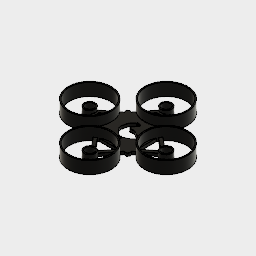
tiny-whoop-redesign (Autodesk Fusion 360 design; units mm, degrees)
Autodesk Fusion 360 part; units mm, degrees
note: some values were not read from the file. Chosen so that the rebuilt part matches the saved one: which bodies a step acts on; which face or edge a step refers to; a direction. Set by a fixed rule: which sketch regions a step uses.
sketch "Sketch1" plane through (0, 0, 0) normal (0, 1, 0) x (1, 0, 0)
  line L0 (-13.5, -13.5) -> (13.5, -13.5)
  line L1 (13.5, -13.5) -> (13.5, 13.5)
  line L2 (13.5, 13.5) -> (-13.5, 13.5)
  line L3 (-13.5, 13.5) -> (-13.5, -13.5)
  line L4 (-13.5, -13.5) -> (13.5, 13.5) construction
  line L5 (13.5, -13.5) -> (-13.5, 13.5) construction
  circle A0 centre (0, 30.8) radius 16.3
  circle A1 centre (0, 30.8) radius 3.5
  circle A2 centre (-13.5, 13.5) radius 2
  line L6 (0, 30.8) -> (13.5, 13.5)
  line L7 (0, 30.8) -> (-13.5, 13.5)
  dimension "d1" = 27
  dimension "d4" = 7
  dimension "d5" = 4
  dimension "d21" = 17.3
  dimension "d22" = 32.6
  dimension "d23" = 27
  measures "d1" distance of L0.end L1.end
  measures "d4" diameter of A1
  measures "d5" diameter of A2
  measures "d21" distance of L2 A0.centre
  measures "d22" diameter of A0
  measures "d23" distance of L1 L3
surface "Extrude1" add extruded along (0, 1, 0) between 0 and 10 path "Sketch1" along A0 makes body 1
surface "Extrude2" add extruded along (0, 1, 0) between 0 and 5 path "Sketch1" along A1 separate body makes body 2
extrude "Extrude3" add sketch "Sketch1" along normal blind 2.5 separate body contours L2 A0 A2 L6 L7 | L2 A2 L7 | A0 A1 L6 L7 picked at (6.7383, 20.8692) makes body 3
shell "Shell1" thickness 2.5 removed faces 2 at (-0.0858, 2.5, -21.0695) at (-0.0858, 0, -21.0695) on bodies 3
thicken "Thicken1" add thickness -1 1 faces at (16.2797, 6.6667, -29.9875) separate body on bodies 1 makes body 4
thicken "Thicken2" add thickness -1 1 faces at (3.4956, 3.3333, -30.6255) separate body on bodies 2 makes body 5
delete_body "RemoveBody1" bodies 2
delete_body "RemoveBody2" bodies 1
extrude "Extrude4" add sketch "Sketch1" along normal blind 2.5 contours L3 A2 L7 | L2 L3 A2 bodies 3
pattern_circular "C-Pattern1" count 4 over 360 about axis through (0, 1.75, 0) along (0, 1, 0) of bodies 4 5 3 makes body 6 at (-14.3333, 2.5, 2.126) makes body 7 at (2.126, 2.5, 14.3333) makes body 8 at (14.3333, 2.5, -2.126) makes body 9 at (-30.5757, 3.3333, -4.4944) makes body 10 at (-4.4944, 3.3333, 30.5757) makes body 11 at (30.5757, 3.3333, 4.4944) makes body 12 at (-29.9377, 6.6667, -17.2785) makes body 13 at (-17.2785, 6.6667, 29.9377) makes body 14 at (29.9377, 6.6667, 17.2785)
extrude "Extrude5" add sketch "Sketch1" along normal blind 2.5 contours L0 L1 L2 L3 A2 bodies 4 5 9 10 11 3 6 7 8 12 13 14
sketch "Sketch2" plane through (0, 0, 0) normal (0, -1, 0) x (1, 0, 0)
  line L0 (17.1612, 10.643) -> (15.0767, 12.2696)
  arc A0 (15.0767, 12.2696) -> (12.2696, 15.0767) centre (13.5, 13.5) ccw
  line L1 (12.2696, 15.0767) -> (10.643, 17.1612)
  arc A1 (10.643, 17.1612) -> (-10.643, 17.1612) centre (0, 30.8) ccw
  line L2 (-10.643, 17.1612) -> (-12.2696, 15.0767)
  arc A2 (-12.2696, 15.0767) -> (-15.0767, 12.2696) centre (-13.5, 13.5) ccw
  line L3 (-15.0767, 12.2696) -> (-17.1612, 10.643)
  arc A3 (-17.1612, 10.643) -> (-17.1612, -10.643) centre (-30.8, 0) ccw
  line L4 (-17.1612, -10.643) -> (-15.0767, -12.2696)
  arc A4 (-15.0767, -12.2696) -> (-12.2696, -15.0767) centre (-13.5, -13.5) ccw
  line L5 (-12.2696, -15.0767) -> (-10.643, -17.1612)
  arc A5 (-10.643, -17.1612) -> (10.643, -17.1612) centre (0, -30.8) ccw
  line L6 (10.643, -17.1612) -> (12.2696, -15.0767)
  arc A6 (12.2696, -15.0767) -> (15.0767, -12.2696) centre (13.5, -13.5) ccw
  line L7 (15.0767, -12.2696) -> (17.1612, -10.643)
  arc A7 (17.1612, -10.643) -> (17.1612, 10.643) centre (30.8, 0) ccw
  line L8 (16.5636, 7.9382) -> (24.9619, 1.3846)
  arc A8 (24.9619, 1.3846) -> (24.9619, -1.3846) centre (30.8, 0) ccw
  line L9 (24.9619, -1.3846) -> (16.5636, -7.9382)
  arc A9 (16, -6.8301) -> (16.5636, -7.9382) centre (30.8, 0) ccw
  line L10 (16, -6.8301) -> (16, 6.8301)
  arc A10 (16.5636, 7.9382) -> (16, 6.8301) centre (30.8, 0) ccw
  arc A11 (10.0278, 17.9496) -> (-10.0278, 17.9496) centre (0, 30.8) ccw
  line L11 (10.0278, 17.9496) -> (2.1532, 28.0407)
  arc A12 (-2.1532, 28.0407) -> (2.1532, 28.0407) centre (0, 30.8) ccw
  line L12 (-2.1532, 28.0407) -> (-10.0278, 17.9496)
  line L13 (-16.5636, -7.9382) -> (-24.9619, -1.3846)
  arc A13 (-24.9619, -1.3846) -> (-24.9619, 1.3846) centre (-30.8, 0) ccw
  line L14 (-24.9619, 1.3846) -> (-16.5636, 7.9382)
  arc A14 (-16, 6.8301) -> (-16.5636, 7.9382) centre (-30.8, 0) ccw
  line L15 (-16, 6.8301) -> (-16, -6.8301)
  arc A15 (-16.5636, -7.9382) -> (-16, -6.8301) centre (-30.8, 0) ccw
  arc A16 (-6.8301, -16) -> (-7.9382, -16.5636) centre (0, -30.8) ccw
  line L16 (-6.8301, -16) -> (6.8301, -16)
  arc A17 (7.9382, -16.5636) -> (6.8301, -16) centre (0, -30.8) ccw
  line L17 (7.9382, -16.5636) -> (1.3846, -24.9619)
  arc A18 (1.3846, -24.9619) -> (-1.3846, -24.9619) centre (0, -30.8) ccw
  line L18 (-1.3846, -24.9619) -> (-7.9382, -16.5636)
  line L19 (-10.0278, -17.9496) -> (-2.1532, -28.0407)
  arc A19 (2.1532, -28.0407) -> (-2.1532, -28.0407) centre (0, -30.8) ccw
  line L20 (2.1532, -28.0407) -> (10.0278, -17.9496)
  arc A20 (-10.0278, -17.9496) -> (10.0278, -17.9496) centre (0, -30.8) ccw
  arc A21 (-17.9496, 10.0278) -> (-17.9496, -10.0278) centre (-30.8, 0) ccw
  line L21 (-17.9496, 10.0278) -> (-28.0407, 2.1532)
  arc A22 (-28.0407, -2.1532) -> (-28.0407, 2.1532) centre (-30.8, 0) ccw
  line L22 (-28.0407, -2.1532) -> (-17.9496, -10.0278)
  line L23 (-7.9382, 16.5636) -> (-1.3846, 24.9619)
  arc A23 (-1.3846, 24.9619) -> (1.3846, 24.9619) centre (0, 30.8) ccw
  line L24 (1.3846, 24.9619) -> (7.9382, 16.5636)
  arc A24 (6.8301, 16) -> (7.9382, 16.5636) centre (0, 30.8) ccw
  line L25 (6.8301, 16) -> (-6.8301, 16)
  arc A25 (-7.9382, 16.5636) -> (-6.8301, 16) centre (0, 30.8) ccw
  arc A26 (17.9496, -10.0278) -> (17.9496, 10.0278) centre (30.8, 0) ccw
  line L26 (17.9496, -10.0278) -> (28.0407, -2.1532)
  arc A27 (28.0407, 2.1532) -> (28.0407, -2.1532) centre (30.8, 0) ccw
  line L27 (28.0407, 2.1532) -> (17.9496, 10.0278)
  spline S0 degree 5 poles (-2.1666, -3.1902) (-2.2131, -3.2344) (-2.2807, -3.3362) (-2.3073, -3.5283) (-2.2123, -3.8513) (-1.9615, -4.3155) (-1.6699, -4.7852) (-1.3964, -5.2241) (-1.1501, -5.6233) (-0.9149, -5.9884) (-0.6643, -6.3303) (-0.3814, -6.6536) (-0.0723, -6.9502) (0.2427, -7.212) (0.5353, -7.44) (0.7768, -7.6596) (0.9424, -7.9138) (1.0132, -8.2368) (0.9784, -8.6265) (0.8354, -9.0411) (0.5869, -9.4231) (0.2388, -9.7158) (-0.2025, -9.884) (-0.7286, -9.9113) (-1.3271, -9.795) (-1.9806, -9.5432) (-2.6636, -9.1699) (-3.3446, -8.6932) (-3.9906, -8.1336) (-4.5708, -7.5131) (-5.0603, -6.8538) (-5.445, -6.1765) (-5.7243, -5.4997) (-5.9167, -4.838) (-6.0522, -4.2019) (-6.1638, -3.5974) (-6.2798, -3.0259) (-6.416, -2.4838) (-6.5658, -1.9619) (-6.6995, -1.4465) (-6.777, -0.9226) (-6.758, -0.3764) (-6.6122, 0.2015) (-6.3322, 0.8132) (-5.9305, 1.4534) (-5.4324, 2.1115) (-4.8694, 2.7725) (-4.2726, 3.4186) (-3.6662, 4.0302) (-3.0606, 4.5878) (-2.4472, 5.0728) (-1.8059, 5.4681) (-1.1109, 5.7582) (-0.337, 5.9299) (0.5338, 5.9725) (1.5068, 5.8782) (2.5667, 5.6426) (3.6785, 5.2653) (4.7946, 4.7507) (5.8602, 4.109) (6.8204, 3.3572) (7.6253, 2.5197) (8.2363, 1.6294) (8.6327, 0.7288) (8.8165, -0.1298) (8.8216, -0.8816) (8.7036, -1.4593) (8.5198, -1.8118) (8.313, -1.9188) (8.0914, -1.8089) (7.8167, -1.5707) (7.4396, -1.3139) (6.9288, -1.1376) (6.3046, -1.0941) (5.6194, -1.1979) (4.9387, -1.4336) (4.3204, -1.7654) (3.7979, -2.145) (3.3545, -2.5209) (2.9336, -2.8453) (2.4654, -3.0801) (1.8893, -3.2034) (1.1766, -3.2154) (0.358, -3.1463) (-0.488, -3.0483) (-1.2626, -2.9819) (-1.747, -2.9997) (-2.0017, -3.071) (-2.1201, -3.146) (-2.1666, -3.1902) knots 0 0 0 0 0 0 0.01176471 0.02352941 0.03529412 0.04705882 0.05882353 0.07058824 0.08235294 0.09411765 0.10588235 0.11764706 0.12941176 0.14117647 0.15294118 0.16470588 0.17647059 0.18823529 0.2 0.21176471 0.22352941 0.23529412 0.24705882 0.25882353 0.27058824 0.28235294 0.29411765 0.30588235 0.31764706 0.32941176 0.34117647 0.35294118 0.36470588 0.37647059 0.38823529 0.4 0.41176471 0.42352941 0.43529412 0.44705882 0.45882353 0.47058824 0.48235294 0.49411765 0.50588235 0.51764706 0.52941176 0.54117647 0.55294118 0.56470588 0.57647059 0.58823529 0.6 0.61176471 0.62352941 0.63529412 0.64705882 0.65882353 0.67058824 0.68235294 0.69411765 0.70588235 0.71764706 0.72941176 0.74117647 0.75294118 0.76470588 0.77647059 0.78823529 0.8 0.81176471 0.82352941 0.83529412 0.84705882 0.85882353 0.87058824 0.88235294 0.89411765 0.90588235 0.91764706 0.92941176 0.94117647 0.95294118 0.96470588 0.97647059 0.98823529 1 1 1 1 1 1
  line L28 (-2.316, -9.3468) -> (-2.5138, -10.5027)
  line L29 (-2.5138, -10.5027) -> (-1.6191, -9.6681)
  line L30 (-0.743, 10.2464) -> (-0.1832, 5.9127)
  line L31 (-0.743, 10.2464) -> (-1.6827, 10.7991)
  line L32 (-1.6827, 10.7991) -> (-1.8453, 10.5227)
  line L33 (-1.8453, 10.5227) -> (-2.0079, 10.2464)
  line L34 (-2.0079, 10.2464) -> (-1.5408, 10.3846)
  line L35 (-1.5408, 10.3846) -> (-1.0317, 10.1717)
  line L36 (-1.0317, 10.1717) -> (-0.918, 5.7789)
  line L37 (0.6389, 5.9355) -> (1.6007, 8.6985)
  line L38 (1.6007, 8.6985) -> (1.7894, 10.9793)
  line L39 (1.7894, 10.9793) -> (1.1198, 11.5623)
  line L40 (1.1198, 11.5623) -> (1.3026, 11.7722)
  line L41 (1.3026, 11.7722) -> (1.8303, 11.3126)
  line L42 (1.8303, 11.3126) -> (2.0304, 11.5424)
  line L43 (2.0304, 11.5424) -> (2.2412, 11.3589)
  line L44 (2.2412, 11.3589) -> (2.0304, 10.9254)
  line L45 (2.0304, 10.9254) -> (1.9304, 8.568)
  line L46 (1.9304, 8.568) -> (1.8125, 5.7917)
  line L47 (8.6687, 0.4386) -> (10.4063, -1.1083)
  line L48 (7.395, -1.3282) -> (9.3462, -3.04)
  line L49 (9.8991, -1.2046) -> (9.5717, -1.5059)
  line L50 (9.4539, -2.0166) -> (9.1527, -2.3702)
  spline S1 degree 2 poles (9.8991, -1.2046) (10.5278, -1.5059) (10.4063, -1.1083) knots 0 0 0 0.088746 0.088746 0.088746 weights 1 3 1
  spline S2 degree 2 poles (9.5717, -1.5059) (10.3051, -2.3571) (9.4539, -2.0166) knots 0 0 0 0.156372 0.156372 0.156372 weights 1 3 1
  spline S3 degree 2 poles (9.1527, -2.3702) (9.8991, -3.2215) (9.3462, -3.04) knots 0 0 0 0.132281 0.132281 0.132281 weights 1 3 1
  point P0 (-1.7712, -4.6196)
  point P1 (-0.7068, -6.2619)
  point P2 (0.3881, -7.3264)
  point P3 (0.9659, -8.0867)
  point P4 (0.5402, -9.4248)
  point P5 (-1.6191, -9.6681)
  point P6 (-5.4512, -6.1099)
  point P7 (-6.3635, -2.7036)
  point P8 (-6.6981, -0.2098)
  point P9 (-3.7631, 3.9228)
  point P10 (0.9821, 5.9127)
  point P11 (8.6687, 0.4386)
  point P12 (8.34, -1.8623)
  point P13 (7.395, -1.3282)
  point P14 (4.1491, -1.9034)
  point P15 (1.6839, -3.1902)
extrude "Extrude6" cut sketch "Sketch2" against normal blind 3 contours S0 | S0 L28 L29 | S0 L47 L48 L49 L50 S1 S2 S3 | S0 L30 L31 L32 L33 L34 L35 L36 | S0 L37 L38 L39 L40 L41 L42 L43 L44 L45 L46 bodies 4
combine "Combine2" operation add target body 4 tool bodies 9 5 10 11
